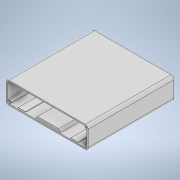
# Autodesk Inventor part: case_dummy
Saved by Autodesk Inventor 2021 (Build 250183000, 183)
## iProperties
Created: 2025-12-27
Part Number: case_dummy
Material: Generic
Document SubType Name: Modeling
Designer: Toby
Density: 1 g/cm^3
Appearance: Default
Author: Toby
Autodesk Inventor part; units mm, degrees
ref_plane "YZ Plane" through (0, 0, 0) normal (1, 0, 0) x (0, 1, 0)
ref_plane "XZ Plane" through (0, 0, 0) normal (0, 1, 0) x (-1, 0, 0)
ref_plane "XY Plane" through (0, 0, 0) normal (0, 0, 1) x (1, 0, 0)
sketch "Sketch1" plane through (0, 0, 0) normal (0, 0, 1) x (1, 0, 0)
  line L0 (-62.25, 16.5) -> (62.25, 16.5)
  line L1 (62.25, 16.5) -> (62.25, -16.5)
  line L2 (62.25, -16.5) -> (-62.25, -16.5)
  line L3 (-62.25, -16.5) -> (-62.25, 16.5)
  line L4 (-60.25, 14.5) -> (60.25, 14.5)
  line L5 (60.25, 14.5) -> (60.25, -14.5)
  line L6 (60.25, -14.5) -> (-60.25, -14.5)
  line L7 (-60.25, -14.5) -> (-60.25, 14.5)
  point P0 (0, 0)
  dimension "d0" = 124.5
  dimension "d1" = 62.25
  dimension "d2" = 120.5
  dimension "d3" = 60.25
  dimension "d4" = 33
  dimension "d5" = 29
  dimension "d6" = 16.5
  dimension "d7" = 14.5
  constraints: 16 end point, 4 parallel, 2 horizontal, 2 perpendicular
  measures "d0" distance of L1.end L2.end
  measures "d1" distance from line of point (0, 0) L3
  measures "d2" distance between parallel lines of L5 L7
  measures "d3" distance from line of point (0, 0) L7
  measures "d4" distance between parallel lines of L2 L0
  measures "d5" distance between parallel lines of L6 L4
  measures "d6" distance from line of point (0, 0) L0
  measures "d7" distance from line of point (0, 0) L4
extrude "Extrusion1" add sketch "Sketch1" against normal blind 130
sketch "Sketch2" plane through (0, 0, 0) normal (0, 0, 1) x (1, 0, 0)
  line L0 (60.25, -14.5) -> (-60.25, -14.5) projected
  line L1 (-15.935, -14.5) -> (15.935, -14.5)
  line L2 (15.935, -14.5) -> (15.935, -10.95)
  line L3 (15.935, -10.95) -> (-15.935, -10.95)
  line L4 (-15.935, -10.95) -> (-15.935, -14.5)
  point P0 (0, 0)
  dimension "d10" = 31.87
  dimension "d11" = 15.935
  dimension "d12" = 3.55
  constraints: 8 end point, 2 parallel, 1 horizontal, 1 perpendicular, 1 point on line
  measures "d10" distance of L2.end L3.end
  measures "d11" distance from line of point (0, 0) L4
  measures "d12" distance between parallel lines of L0 L3
extrude "Extrusion2" add sketch "Sketch2" against normal blind 130
chamfer "Chamfer1" distance 3.55 angle 45 2 edges at (15.935, -14.5, -65) (-15.935, -14.5, -65)
sketch "Sketch3" plane through (0, 0, 0) normal (0, 0, 1) x (1, 0, 0)
  line L0 (-19.485, -14.5) -> (-60.25, -14.5) projected
  line L1 (-45.4675, -14.5) -> (-34.2675, -14.5)
  line L2 (-34.2675, -14.5) -> (-34.2675, -14.05)
  line L3 (-34.2675, -14.05) -> (-45.4675, -14.05)
  line L4 (-45.4675, -14.05) -> (-45.4675, -14.5)
  line L5 (-60.25, 14.5) -> (-60.25, -14.5) projected
  point P0 (0, 0)
  point P1 (-60.25, -14.5)
  dimension "d18" = 40.765
  dimension "d19" = 11.2
  dimension "d20" = 0.45
  dimension "d21" = 14.7825
  dimension "d22" = 14.7825
  constraints: 8 end point, 2 coincident, 2 parallel, 1 horizontal, 1 perpendicular, 1 point on line
  measures "d18" distance of L0.start point (-60.25, -14.5)
  measures "d19" distance of L2.end L3.end
  measures "d20" distance between parallel lines of L0 L3
  measures "d21" distance of L0.start L1.end
  measures "d22" distance of L0.end L1.start
extrude "Extrusion3" add sketch "Sketch3" against normal blind 130
chamfer "Chamfer2" distance 0.45 angle 45 2 edges at (-45.4675, -14.5, -65) (-34.2675, -14.5, -65)
sketch "Sketch4" plane through (0, 0, 0) normal (0, 0, 1) x (1, 0, 0)
  line L0 (60.25, -14.5) -> (19.485, -14.5) projected
  line L1 (34.2675, -14.5) -> (45.4675, -14.5)
  line L2 (45.4675, -14.5) -> (45.4675, -14.05)
  line L3 (45.4675, -14.05) -> (34.2675, -14.05)
  line L4 (34.2675, -14.05) -> (34.2675, -14.5)
  point P0 (0, 0)
  dimension "d28" = 11.2
  dimension "d29" = 0.45
  dimension "d30" = 14.7825
  constraints: 8 end point, 2 parallel, 1 horizontal, 1 perpendicular, 1 point on line
  measures "d28" distance of L2.end L3.end
  measures "d29" distance between parallel lines of L0 L3
  measures "d30" horizontal distance of L0.start L2.end
extrude "Extrusion4" add sketch "Sketch4" against normal blind 130
chamfer "Chamfer3" distance 0.45 angle 45 2 edges at (34.2675, -14.5, -65) (45.4675, -14.5, -65)
sketch "Sketch5" plane through (0, 0, 0) normal (0, 0, 1) x (1, 0, 0)
  circle A0 centre (-57.8, 12.05) radius 2
  circle A1 centre (57.8, 12.05) radius 2
  line L0 (62.25, -16.5) -> (62.25, 16.5) projected
  line L1 (62.25, 16.5) -> (-62.25, 16.5) projected
  line L2 (-62.25, 16.5) -> (-62.25, -16.5) projected
  line L3 (-60.25, 14.5) -> (-60.25, -14.5) projected
  line L4 (-57.8, 10.05) -> (-60.25, 10.05)
  line L5 (-60.25, 10.05) -> (-60.25, 14.5)
  line L6 (-60.25, 14.5) -> (-57.8, 14.5)
  line L7 (-57.8, 14.5) -> (-57.8, 10.05)
  line L8 (-57.8, 14.5) -> (-57.2, 14.5)
  line L9 (-57.2, 14.5) -> (-57.2, 13.9579)
  line L10 (-57.2, 13.9579) -> (-57.8, 13.9579)
  line L11 (-57.8, 13.9579) -> (-57.8, 14.5)
  line L12 (60.25, 14.5) -> (-60.25, 14.5) projected
  line L13 (60.25, 14.5) -> (57.8, 14.5)
  line L14 (57.8, 14.5) -> (57.8, 10.05)
  line L15 (57.8, 10.05) -> (60.25, 10.05)
  line L16 (60.25, 10.05) -> (60.25, 14.5)
  line L17 (57.8, 14.5) -> (57.2, 14.5)
  line L18 (57.2, 14.5) -> (57.2, 13.9579)
  line L19 (57.2, 13.9579) -> (57.8, 13.9579)
  line L20 (57.8, 13.9579) -> (57.8, 14.5)
  circle A2 centre (-57.8, -12.05) radius 2
  circle A3 centre (57.8, -12.05) radius 2
  line L21 (-62.25, -16.5) -> (62.25, -16.5) projected
  line L22 (-57.8, -10.05) -> (-60.25, -10.05)
  line L23 (-60.25, -10.05) -> (-60.25, -14.5)
  line L24 (-60.25, -14.5) -> (-57.8, -14.5)
  line L25 (-57.8, -14.5) -> (-57.8, -10.05)
  line L26 (60.25, 14.5) -> (60.25, -14.5) projected
  line L27 (57.8, -10.05) -> (60.25, -10.05)
  line L28 (60.25, -10.05) -> (60.25, -14.5)
  line L29 (60.25, -14.5) -> (57.8, -14.5)
  line L30 (57.8, -14.5) -> (57.8, -10.05)
  line L31 (57.2, -13.9579) -> (57.8, -13.9579)
  line L32 (57.8, -13.9579) -> (57.8, -14.5)
  line L33 (57.8, -14.5) -> (57.2, -14.5)
  line L34 (57.2, -14.5) -> (57.2, -13.9579)
  line L35 (-57.8, -14.5) -> (-57.0401, -14.5)
  line L36 (-57.0401, -14.5) -> (-57.0401, -13.9)
  line L37 (-57.0401, -13.9) -> (-57.8, -13.9)
  line L38 (-57.8, -13.9) -> (-57.8, -14.5)
  point P0 (0, 0)
  point P1 (-55.8, 12.05)
  point P2 (55.8, 12.05)
  dimension "d36" = 115.6
  dimension "d37" = 4.45
  dimension "d38" = 4.45
  dimension "d39" = 4.45
  dimension "d40" = 4.45
  dimension "d41" = 111.6
  dimension "d42" = 4
  dimension "d43" = 4
  dimension "d44" = 0.6
  dimension "d45" = 4.45
  dimension "d46" = 4.45
  dimension "d47" = 0.6
  dimension "d48" = 4
  dimension "d49" = 4.45
  dimension "d50" = 4.45
  dimension "d51" = 4.45
  dimension "d52" = 4.45
  dimension "d53" = 0.6
  dimension "d54" = 4.45
  dimension "d55" = 4
  dimension "d56" = 0.6
  constraints: 64 end point, 16 parallel, 10 point on circle, 8 horizontal, 8 perpendicular, 4 centre point, 1 point on line
  measures "d36" distance of A0.centre A1.centre
  measures "d37" distance from line of L0 A1.centre
  measures "d38" distance from line of L1 A1.centre
  measures "d39" distance from line of L2 A0.centre
  measures "d40" distance from line of L1 A0.centre
  measures "d41" distance of A1.start A0.start
  measures "d42" diameter of A0
  measures "d43" diameter of A1
  measures "d44" distance of L9.end L10.end
  measures "d45" distance between parallel lines of L6 L4
  measures "d46" distance of L13.end L14.end
  measures "d47" distance of L18.end L19.end
  measures "d48" diameter of A2
  measures "d49" distance from line of L21 A3.centre
  measures "d50" distance from line of L0 A3.centre
  measures "d51" distance from line of L2 A2.centre
  measures "d52" distance from line of L21 A2.centre
  measures "d53" distance of L31.start L31.end
  measures "d54" distance of L29.end L27.start
  measures "d55" diameter of A3
  measures "d56" distance of L35.end L36.end
extrude "Extrusion5" add sketch "Sketch5" against normal blind 130 contours A0 L7 L10 | L22 A2 L25 L24 L3 | L26 L29 L30 A3 L27 | L12 L14 A1 L18 | L10 L7 A0 | A0 L7 L8 L9 | L4 L3 L6 L7 A0 | A0 L7 | L12 L16 L15 A1 L14 | L19 L14 A1 | A1 L14 L19 | L25 A2 | A2 L37 L25 | A1 L14 | L25 A2 L36 L35 | L25 L37 A2 | L30 L31 A3 | A3 L30 | L33 L34 A3 L30 | L31 L30 A3
sketch "Sketch6" plane through (0, 0, 0) normal (0, 0, 1) x (1, 0, 0)
  arc A0 (-57.8, 10.05) -> (-57.2, 13.9579) centre (-57.8, 12.05) ccw projected
  arc A1 (-57.0401, -13.9) -> (-57.8, -10.05) centre (-57.8, -12.05) ccw projected
  arc A2 (57.8, -10.05) -> (57.2, -13.9579) centre (57.8, -12.05) ccw projected
  arc A3 (57.2, 13.9579) -> (57.8, 10.05) centre (57.8, 12.05) ccw projected
  circle A4 centre (-57.8, 12.05) radius 1
  circle A5 centre (-57.8, -12.05) radius 1
  circle A6 centre (57.8, -12.05) radius 1
  circle A7 centre (57.8, 12.05) radius 1
  point P0 (0, 0)
  dimension "d59" = 2
  dimension "d60" = 2
  dimension "d61" = 2
  dimension "d62" = 2
  constraints: 8 coincident, 4 centre point
  measures "d59" diameter of A4
  measures "d60" diameter of A5
  measures "d61" diameter of A6
  measures "d62" diameter of A7
extrude "Extrusion6" cut sketch "Sketch6" against normal blind 130
fillet "Fillet1" radius 4.45 4 edges at (-62.25, 16.5, -65) (-62.25, -16.5, -65) (62.25, -16.5, -65) (62.25, 16.5, -65)
sketch "Sketch7" plane through (0, 0, 0) normal (0, 0, 1) x (1, 0, 0)
  line L0 (-60.25, 14.5) -> (60.25, 14.5)
  line L1 (60.25, 14.5) -> (60.25, -14.5)
  line L2 (60.25, -14.5) -> (-60.25, -14.5)
  line L3 (-60.25, -14.5) -> (-60.25, 14.5)
  line L4 (-57.2, 14.5) -> (57.2, 14.5) projected
  line L5 (60.25, 10.05) -> (60.25, -10.05) projected
  line L6 (33.8175, -14.5) -> (19.485, -14.5) projected
  line L7 (-60.25, -10.05) -> (-60.25, 10.05) projected
  arc A0 (-57.8, 10.05) -> (-57.2, 13.9579) centre (-57.8, 12.05) ccw projected
  circle A1 centre (-57.8, 12.05) radius 2.45
  arc A2 (-57.0401, -13.9) -> (-57.8, -10.05) centre (-57.8, -12.05) ccw projected
  circle A3 centre (-57.8, -12.05) radius 2.45
  circle A4 centre (57.8, -12.05) radius 1 projected
  circle A5 centre (57.8, -12.05) radius 2.45
  circle A6 centre (57.8, 12.05) radius 1 projected
  circle A7 centre (57.8, 12.05) radius 2.45
  point P0 (0, 0)
  point P1 (57.8, 14.5)
  point P2 (-57.8, 14.5)
  point P3 (-60.25, 12.05)
  point P4 (-60.25, -12.05)
  point P5 (-57.8, -14.5)
  point P6 (57.8, -14.5)
  point P7 (60.25, -12.05)
  point P8 (60.25, 12.05)
  constraints: 8 end point, 4 centre point, 4 coincident, 4 collinear, 4 tangent, 2 parallel, 1 horizontal, 1 perpendicular
extrude "Extrusion7" cut sketch "Sketch7" against normal blind 1.5 contours L0 A7 L1 A5 L2 A3 L3 A1 | A1 | A7 | A3 | A5 | A4 | A6
sketch "Sketch8" plane through (0, 0, -130) normal (0, 0, -1) x (-1, 0, 0)
  line L0 (-60.25, 14.5) -> (60.25, 14.5)
  line L1 (60.25, 14.5) -> (60.25, -14.5)
  line L2 (60.25, -14.5) -> (-60.25, -14.5)
  line L3 (-60.25, -14.5) -> (-60.25, 14.5)
  line L4 (-57.2, 14.5) -> (57.2, 14.5) projected
  line L5 (60.25, 10.05) -> (60.25, -10.05) projected
  line L6 (33.8175, -14.5) -> (19.485, -14.5) projected
  line L7 (-60.25, -10.05) -> (-60.25, 10.05) projected
  circle A0 centre (-57.8, 12.05) radius 1 projected
  circle A1 centre (-57.8, 12.05) radius 2.45
  line L8 (57.8, 14.5) -> (-57.8, 14.5) projected
  circle A2 centre (-57.8, -12.05) radius 1 projected
  circle A3 centre (-57.8, -12.05) radius 2.45
  circle A4 centre (57.8, -12.05) radius 1 projected
  line L9 (-57.8, -14.5) -> (57.8, -14.5) projected
  circle A5 centre (57.8, -12.05) radius 2.45
  circle A6 centre (57.8, 12.05) radius 1 projected
  circle A7 centre (57.8, 12.05) radius 2.45
  point P0 (0, 0)
  point P1 (-60.25, 12.05)
  point P2 (-60.25, -12.05)
  point P3 (-57.8, -14.5)
  point P4 (60.25, -12.05)
  point P5 (60.25, 12.05)
  constraints: 8 end point, 4 coincident, 4 collinear, 3 centre point, 3 tangent, 2 parallel, 1 horizontal, 1 perpendicular, 3 other
extrude "Extrusion8" cut sketch "Sketch8" against normal blind 1.5 contours L0 A7 L1 A5 L2 A3 L3 A1 | A1 | A7 | A3 | A5 | A0 | A2 | A4 | A6
body "Solid1"
